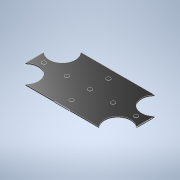
# Autodesk Inventor part: FORS phone case- base
Saved by Autodesk Inventor 2021 (Build 250183000, 183)
## iProperties
Created: 2020-06-20
Part Number: FORS phone case- base
Material: Generic
Document SubType Name: Modeling
Designer: david
Density: 1 g/cm^3
Appearance: Glossy - Black
Author: david
Autodesk Inventor part; units mm, degrees
ref_plane "YZ Plane" through (0, 0, 0) normal (1, 0, 0) x (0, 1, 0)
ref_plane "XZ Plane" through (0, 0, 0) normal (0, 1, 0) x (-1, 0, 0)
ref_plane "XY Plane" through (0, 0, 0) normal (0, 0, 1) x (1, 0, 0)
sketch "Sketch1" plane through (0, 0, 0) normal (0, 1, 0) x (-1, 0, 0)
  line L0 (37.5811, -104.7549) -> (37.5811, -130.1549)
  line L1 (62.9811, -155.5549) -> (164.5811, -155.5549)
  line L2 (189.9811, -130.1549) -> (189.9811, -104.7549)
  arc A0 (62.9811, -155.5549) -> (37.5811, -130.1549) centre (50.2811, -142.8549) ccw
  arc A1 (189.9811, -130.1549) -> (164.5811, -155.5549) centre (177.2811, -142.8549) ccw
  arc A2 (164.5811, -79.3549) -> (189.9811, -104.7549) centre (177.2811, -92.0549) ccw
  arc A3 (37.5811, -104.7549) -> (62.9811, -79.3549) centre (50.2811, -92.0549) ccw
  line L3 (164.5811, -79.3549) -> (62.9811, -79.3549)
  point P0 (0, 0)
  dimension "d4" = 17.9605
  dimension "d11" = 17.9605
  dimension "d16" = 25.4
  dimension "d17" = 17.9605
  dimension "d18" = 25.4
  dimension "d19" = 101.6
  dimension "d20" = 17.9605
  constraints: 8 end point, 8 point on circle, 4 centre point, 2 parallel, 1 horizontal, 1 perpendicular
  measures "d4" radius of A0
  measures "d11" radius of A1
  measures "d16" distance of L0.end L0.start
  measures "d17" radius of A3
  measures "d18" distance of L2.start L2.end
  measures "d19" distance of L1.start L1.end
  measures "d20" radius of A2
extrude "Extrusion1" add sketch "Sketch1" along normal blind 1.5875
sketch "Sketch2" plane through (0, 1.5875, 0) normal (0, 1, 0) x (1, 0, 0)
  circle A0 centre (-113.7811, 117.4549) radius 2.7481
  line L0 (-62.9811, 155.5549) -> (-164.5811, 155.5549) projected
  line L1 (-37.5811, 104.7549) -> (-37.5811, 130.1549) projected
  circle A1 centre (-145.5311, 117.4549) radius 2.7481
  circle A2 centre (-177.2811, 117.4549) radius 2.7481
  circle A3 centre (-82.0311, 117.4549) radius 2.7481
  circle A4 centre (-50.2811, 117.4549) radius 2.7481
  circle A5 centre (-113.7811, 142.8549) radius 2.7481
  circle A6 centre (-113.7811, 92.0549) radius 2.7481
  point P0 (0, 0)
  dimension "d23" = 38.1
  dimension "d24" = 76.2
  dimension "d27" = 31.75
  dimension "d34" = 31.75
  dimension "d41" = 25.4
  dimension "d48" = 25.4
  constraints: 7 centre point, 2 horizontal, 2 vertical, 12 other
  measures "d23" distance from line of L0 A0.centre
  measures "d24" distance from line of L1 A0.centre
  measures "d27" distance of A0.centre A1.centre
  measures "d34" distance of A0.centre A3.centre
  measures "d41" distance of A0.centre A5.centre
  measures "d48" distance of A0.centre A6.centre
extrude "Extrusion2" add sketch "Sketch2" along normal blind 0.508
sketch "Sketch3" plane through (-189.9811, 0, -130.1549) normal (-1, 0, 0) x (0, 0, 1)
  line L0 (24.5513, 1.3891) -> (4.2313, 1.3891)
  line L1 (4.2313, 1.3891) -> (4.2313, 0.1984)
  line L2 (4.2313, 0.1984) -> (24.5513, 0.1984)
  line L3 (24.5513, 0.1984) -> (24.5513, 1.3891)
  line L4 (0, 0) -> (0, 1.5875) projected
  line L5 (0, 0) -> (25.4, 0) projected
  line L6 (25.4, 0) -> (25.4, 1.5875) projected
  line L7 (0, 1.5875) -> (25.4, 1.5875) projected
  point P0 (130.1549, 0)
  dimension "d55" = 1.5875
  dimension "d56" = 25.4
  dimension "d57" = 1.1906
  dimension "d58" = 0.1984
  dimension "d59" = 20.32
  constraints: 8 end point, 2 parallel, 1 horizontal, 1 perpendicular
  measures "d55" distance of L5.end L6.end
  measures "d56" distance of L4.start L5.end
  measures "d57" distance of L2.end L0.start
  measures "d58" distance between parallel lines of L7 L0
  measures "d59" distance of L1.end L2.end
sketch "Sketch4" plane through (-37.5811, 0, -104.7549) normal (1, 0, 0) x (0, 0, -1)
  line L0 (0, 1.5875) -> (25.4, 1.5875) projected
  line L1 (0, 0) -> (0, 1.5875) projected
  line L2 (25.4, 0) -> (25.4, 1.5875) projected
  line L3 (0.9323, 0.1905) -> (21.2523, 0.1905)
  line L4 (21.2523, 0.1905) -> (21.2523, 1.3843)
  line L5 (21.2523, 1.3843) -> (0.9323, 1.3843)
  line L6 (0.9323, 1.3843) -> (0.9323, 0.1905)
  point P0 (-104.7549, 0)
  dimension "d60" = 20.32
  dimension "d61" = 1.1938
  dimension "d62" = 0.2032
  constraints: 8 end point, 2 parallel, 1 horizontal, 1 perpendicular
  measures "d60" distance of L3.start L3.end
  measures "d61" distance of L3.end L4.end
  measures "d62" distance between parallel lines of L0 L5
extrude "Extrusion3" add sketch "Sketch4" along normal blind 0.508
sketch "Sketch5" plane through (-62.9811, 0, -155.5549) normal (0, 0, -1) x (-1, 0, 0)
  line L0 (101.6, 0) -> (101.6, 1.5875) projected
  line L1 (0, 0) -> (0, 1.5875) projected
  line L2 (40.64, 0.2032) -> (60.96, 0.2032)
  line L3 (60.96, 0.2032) -> (60.96, 1.397)
  line L4 (60.96, 1.397) -> (40.64, 1.397)
  line L5 (40.64, 1.397) -> (40.64, 0.2032)
  line L6 (0, 1.5875) -> (101.6, 1.5875) projected
  line L7 (0, 0) -> (101.6, 0) projected
  point P0 (-62.9811, 0)
  dimension "d65" = 20.32
  dimension "d66" = 40.64
  dimension "d67" = 101.6
  dimension "d68" = 40.64
  dimension "d69" = 1.1938
  dimension "d70" = 0.2032
  dimension "d71" = 0.1905
  constraints: 8 end point, 2 parallel, 1 horizontal, 1 perpendicular
  measures "d65" distance of L3.end L4.end
  measures "d66" distance between parallel lines of L1 L5
  measures "d67" distance of L1.end L0.end
  measures "d68" distance between parallel lines of L3 L0
  measures "d69" distance between parallel lines of L4 L2
  measures "d70" distance between parallel lines of L7 L2
  measures "d71" distance between parallel lines of L6 L4
extrude "Extrusion4" add sketch "Sketch5" along normal blind 0.508 contours L5 L4 L3 L2
extrude "Extrusion5" add sketch "Sketch3" along normal blind 0.508 contours L3 L2 L1 L0
sketch "Sketch6" plane through (-164.5811, 0, -79.3549) normal (0, 0, 1) x (1, 0, 0)
  line L0 (101.6, 0) -> (101.6, 1.5875) projected
  line L1 (0, 0) -> (0, 1.5875) projected
  line L2 (60.96, 0.2032) -> (40.64, 0.2032)
  line L3 (40.64, 0.2032) -> (40.64, 1.397)
  line L4 (40.64, 1.397) -> (60.96, 1.397)
  line L5 (60.96, 1.397) -> (60.96, 0.2032)
  line L6 (0, 0) -> (101.6, 0) projected
  point P0 (164.5811, 0)
  dimension "d76" = 20.32
  dimension "d77" = 1.1938
  dimension "d78" = 0.2032
  dimension "d79" = 40.64
  constraints: 8 end point, 2 parallel, 1 horizontal, 1 perpendicular
  measures "d76" distance of L2.start L2.end
  measures "d77" distance of L4.end L2.start
  measures "d78" distance between parallel lines of L6 L2
  measures "d79" distance between parallel lines of L1 L3
extrude "Extrusion6" add sketch "Sketch6" along normal blind 0.508
equation "\"d57\" = 0.75 * d55"
equation "\"d58\" = -0.5 * d57 + 0.5 * d55"
body "Solid1"
